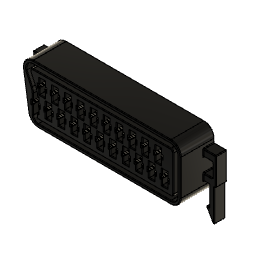
Female SCART connector ST107R-21 (Autodesk Fusion 360 design; units mm, degrees)
Autodesk Fusion 360 part; units mm, degrees
(part 1 of 2)
sketch "Sketch1" plane through (0, 0, 0) normal (0, 1, 0) x (1, 0, 0)
  line L0 (0, 0) -> (47.1, 0)
  line L1 (47.1, 0) -> (47.1, -16.5)
  line L2 (47.1, -16.5) -> (0, -16.5)
  line L3 (0, -16.5) -> (0, 0)
  line L4 (47.1, -8.25) -> (0, -8.25) construction
  line L5 (47.1, -5.71) -> (0, -5.71) construction
  line L6 (47.1, -10.79) -> (0, -10.79) construction
  line L7 (23.3, 0) -> (23.3, -16.5) construction
  line L8 (22.5, -7.81) -> (24.1, -7.81)
  line L9 (24.1, -7.81) -> (24.1, -3.61)
  line L10 (24.1, -3.61) -> (22.5, -3.61)
  line L11 (22.5, -3.61) -> (22.5, -7.81)
  line L12 (5.05, -3.61) -> (3.45, -3.61)
  line L13 (5.05, -7.81) -> (5.05, -3.61)
  line L14 (3.45, -3.61) -> (3.45, -7.81)
  line L15 (3.45, -7.81) -> (5.05, -7.81)
  line L16 (8.86, -3.61) -> (7.26, -3.61)
  line L17 (8.86, -7.81) -> (8.86, -3.61)
  line L18 (7.26, -3.61) -> (7.26, -7.81)
  line L19 (7.26, -7.81) -> (8.86, -7.81)
  line L20 (12.67, -3.61) -> (11.07, -3.61)
  line L21 (12.67, -7.81) -> (12.67, -3.61)
  line L22 (11.07, -3.61) -> (11.07, -7.81)
  line L23 (11.07, -7.81) -> (12.67, -7.81)
  line L24 (16.48, -3.61) -> (14.88, -3.61)
  line L25 (16.48, -7.81) -> (16.48, -3.61)
  line L26 (14.88, -3.61) -> (14.88, -7.81)
  line L27 (14.88, -7.81) -> (16.48, -7.81)
  line L28 (20.29, -3.61) -> (18.69, -3.61)
  line L29 (20.29, -7.81) -> (20.29, -3.61)
  line L30 (18.69, -3.61) -> (18.69, -7.81)
  line L31 (18.69, -7.81) -> (20.29, -7.81)
  line L32 (27.91, -3.61) -> (26.31, -3.61)
  line L33 (27.91, -7.81) -> (27.91, -3.61)
  line L34 (26.31, -3.61) -> (26.31, -7.81)
  line L35 (26.31, -7.81) -> (27.91, -7.81)
  line L36 (31.72, -3.61) -> (30.12, -3.61)
  line L37 (31.72, -7.81) -> (31.72, -3.61)
  line L38 (30.12, -3.61) -> (30.12, -7.81)
  line L39 (30.12, -7.81) -> (31.72, -7.81)
  line L40 (35.53, -3.61) -> (33.93, -3.61)
  line L41 (35.53, -7.81) -> (35.53, -3.61)
  line L42 (33.93, -3.61) -> (33.93, -7.81)
  line L43 (33.93, -7.81) -> (35.53, -7.81)
  line L44 (39.34, -3.61) -> (37.74, -3.61)
  line L45 (39.34, -7.81) -> (39.34, -3.61)
  line L46 (37.74, -3.61) -> (37.74, -7.81)
  line L47 (37.74, -7.81) -> (39.34, -7.81)
  line L48 (43.15, -3.61) -> (41.55, -3.61)
  line L49 (43.15, -7.81) -> (43.15, -3.61)
  line L50 (41.55, -3.61) -> (41.55, -7.81)
  line L51 (41.55, -7.81) -> (43.15, -7.81)
  line L52 (39.34, -7.81) -> (41.55, -7.81) construction
  line L53 (40.445, -7.81) -> (40.445, -14) construction
  line L54 (39.645, -12.89) -> (41.245, -12.89)
  line L55 (41.245, -12.89) -> (41.245, -8.69)
  line L56 (41.245, -8.69) -> (39.645, -8.69)
  line L57 (39.645, -8.69) -> (39.645, -12.89)
  line L58 (37.435, -12.89) -> (37.435, -8.69)
  line L59 (37.435, -8.69) -> (35.835, -8.69)
  line L60 (35.835, -8.69) -> (35.835, -12.89)
  line L61 (35.835, -12.89) -> (37.435, -12.89)
  line L62 (33.625, -12.89) -> (33.625, -8.69)
  line L63 (33.625, -8.69) -> (32.025, -8.69)
  line L64 (32.025, -8.69) -> (32.025, -12.89)
  line L65 (32.025, -12.89) -> (33.625, -12.89)
  line L66 (29.815, -12.89) -> (29.815, -8.69)
  line L67 (29.815, -8.69) -> (28.215, -8.69)
  line L68 (28.215, -8.69) -> (28.215, -12.89)
  line L69 (28.215, -12.89) -> (29.815, -12.89)
  line L70 (26.005, -12.89) -> (26.005, -8.69)
  line L71 (26.005, -8.69) -> (24.405, -8.69)
  line L72 (24.405, -8.69) -> (24.405, -12.89)
  line L73 (24.405, -12.89) -> (26.005, -12.89)
  line L74 (22.195, -12.89) -> (22.195, -8.69)
  line L75 (22.195, -8.69) -> (20.595, -8.69)
  line L76 (20.595, -8.69) -> (20.595, -12.89)
  line L77 (20.595, -12.89) -> (22.195, -12.89)
  line L78 (18.385, -12.89) -> (18.385, -8.69)
  line L79 (18.385, -8.69) -> (16.785, -8.69)
  line L80 (16.785, -8.69) -> (16.785, -12.89)
  line L81 (16.785, -12.89) -> (18.385, -12.89)
  line L82 (14.575, -12.89) -> (14.575, -8.69)
  line L83 (14.575, -8.69) -> (12.975, -8.69)
  line L84 (12.975, -8.69) -> (12.975, -12.89)
  line L85 (12.975, -12.89) -> (14.575, -12.89)
  line L86 (10.765, -12.89) -> (10.765, -8.69)
  line L87 (10.765, -8.69) -> (9.165, -8.69)
  line L88 (9.165, -8.69) -> (9.165, -12.89)
  line L89 (9.165, -12.89) -> (10.765, -12.89)
  line L90 (6.955, -12.89) -> (6.955, -8.69)
  line L91 (6.955, -8.69) -> (5.355, -8.69)
  line L92 (5.355, -8.69) -> (5.355, -12.89)
  line L93 (5.355, -12.89) -> (6.955, -12.89)
  line L94 (0, -16.5) -> (2.5, 0)
  line L95 (22.1, -6.21) -> (24.5, -6.21)
  line L96 (24.5, -6.21) -> (24.5, -5.21)
  line L97 (24.5, -5.21) -> (22.1, -5.21)
  line L98 (22.1, -5.21) -> (22.1, -6.21)
  line L99 (5.45, -5.21) -> (3.05, -5.21)
  line L100 (5.45, -6.21) -> (5.45, -5.21)
  line L101 (3.05, -6.21) -> (5.45, -6.21)
  line L102 (3.05, -5.21) -> (3.05, -6.21)
  line L103 (9.26, -5.21) -> (6.86, -5.21)
  line L104 (9.26, -6.21) -> (9.26, -5.21)
  line L105 (6.86, -6.21) -> (9.26, -6.21)
  line L106 (6.86, -5.21) -> (6.86, -6.21)
  line L107 (13.07, -5.21) -> (10.67, -5.21)
  line L108 (13.07, -6.21) -> (13.07, -5.21)
  line L109 (10.67, -6.21) -> (13.07, -6.21)
  line L110 (10.67, -5.21) -> (10.67, -6.21)
  line L111 (16.88, -5.21) -> (14.48, -5.21)
  line L112 (16.88, -6.21) -> (16.88, -5.21)
  line L113 (14.48, -6.21) -> (16.88, -6.21)
  line L114 (14.48, -5.21) -> (14.48, -6.21)
  line L115 (20.69, -5.21) -> (18.29, -5.21)
  line L116 (20.69, -6.21) -> (20.69, -5.21)
  line L117 (18.29, -6.21) -> (20.69, -6.21)
  line L118 (18.29, -5.21) -> (18.29, -6.21)
  line L119 (28.31, -5.21) -> (25.91, -5.21)
  line L120 (28.31, -6.21) -> (28.31, -5.21)
  line L121 (25.91, -6.21) -> (28.31, -6.21)
  line L122 (25.91, -5.21) -> (25.91, -6.21)
  line L123 (32.12, -5.21) -> (29.72, -5.21)
  line L124 (32.12, -6.21) -> (32.12, -5.21)
  line L125 (29.72, -6.21) -> (32.12, -6.21)
  line L126 (29.72, -5.21) -> (29.72, -6.21)
  line L127 (35.93, -5.21) -> (33.53, -5.21)
  line L128 (35.93, -6.21) -> (35.93, -5.21)
  line L129 (33.53, -6.21) -> (35.93, -6.21)
  line L130 (33.53, -5.21) -> (33.53, -6.21)
  line L131 (39.74, -5.21) -> (37.34, -5.21)
  line L132 (39.74, -6.21) -> (39.74, -5.21)
  line L133 (37.34, -6.21) -> (39.74, -6.21)
  line L134 (37.34, -5.21) -> (37.34, -6.21)
  line L135 (43.55, -5.21) -> (41.15, -5.21)
  line L136 (43.55, -6.21) -> (43.55, -5.21)
  line L137 (41.15, -6.21) -> (43.55, -6.21)
  line L138 (41.15, -5.21) -> (41.15, -6.21)
  line L139 (39.245, -11.29) -> (41.645, -11.29)
  line L140 (41.645, -11.29) -> (41.645, -10.29)
  line L141 (41.645, -10.29) -> (39.245, -10.29)
  line L142 (39.245, -10.29) -> (39.245, -11.29)
  line L143 (35.435, -11.29) -> (37.835, -11.29)
  line L144 (37.835, -10.29) -> (35.435, -10.29)
  line L145 (35.435, -10.29) -> (35.435, -11.29)
  line L146 (37.835, -11.29) -> (37.835, -10.29)
  line L147 (31.625, -11.29) -> (34.025, -11.29)
  line L148 (34.025, -10.29) -> (31.625, -10.29)
  line L149 (31.625, -10.29) -> (31.625, -11.29)
  line L150 (34.025, -11.29) -> (34.025, -10.29)
  line L151 (27.815, -11.29) -> (30.215, -11.29)
  line L152 (30.215, -10.29) -> (27.815, -10.29)
  line L153 (27.815, -10.29) -> (27.815, -11.29)
  line L154 (30.215, -11.29) -> (30.215, -10.29)
  line L155 (24.005, -11.29) -> (26.405, -11.29)
  line L156 (26.405, -10.29) -> (24.005, -10.29)
  line L157 (24.005, -10.29) -> (24.005, -11.29)
  line L158 (26.405, -11.29) -> (26.405, -10.29)
  line L159 (20.195, -11.29) -> (22.595, -11.29)
  line L160 (22.595, -10.29) -> (20.195, -10.29)
  line L161 (20.195, -10.29) -> (20.195, -11.29)
  line L162 (22.595, -11.29) -> (22.595, -10.29)
  line L163 (16.385, -11.29) -> (18.785, -11.29)
  line L164 (18.785, -10.29) -> (16.385, -10.29)
  line L165 (16.385, -10.29) -> (16.385, -11.29)
  line L166 (18.785, -11.29) -> (18.785, -10.29)
  line L167 (12.575, -11.29) -> (14.975, -11.29)
  line L168 (14.975, -10.29) -> (12.575, -10.29)
  line L169 (12.575, -10.29) -> (12.575, -11.29)
  line L170 (14.975, -11.29) -> (14.975, -10.29)
  line L171 (8.765, -11.29) -> (11.165, -11.29)
  line L172 (11.165, -10.29) -> (8.765, -10.29)
  line L173 (8.765, -10.29) -> (8.765, -11.29)
  line L174 (11.165, -11.29) -> (11.165, -10.29)
  line L175 (4.955, -11.29) -> (7.355, -11.29)
  line L176 (7.355, -10.29) -> (4.955, -10.29)
  line L177 (4.955, -10.29) -> (4.955, -11.29)
  line L178 (7.355, -11.29) -> (7.355, -10.29)
  dimension "d15" = 47.1
  dimension "d16" = 16.5
  dimension "d19" = 5.08
  dimension "d20" = 23.8
  dimension "d21" = 1.6
  dimension "d22" = 4.2
  dimension "d25" = 3.81
  dimension "d26" = 0
  dimension "d27" = 4.2
  dimension "d28" = 1.6
  dimension "d31" = -3.81
  dimension "d32" = 0
  dimension "d36" = 1
  dimension "d37" = 2.4
  dimension "d38" = 2.4
  dimension "d39" = 1
  constraint horizontal L0
  constraint vertical L1
  constraint horizontal L2
  constraint vertical L3
  constraint coincident L0.start L3.end
  constraint midpoint L1 L4.start
  constraint midpoint L3 L4.end
  constraint parallel L4 L5
  constraint parallel L4 L6
  constraint symmetric L4 L5 L6
  constraint horizontal L8
  constraint vertical L9
  constraint horizontal L10
  constraint vertical L11
  constraint symmetric L5 L8 L10
  constraint symmetric L7 L9 L11
  constraint midpoint L52 L53.start
  constraint perpendicular L6 L53
  constraint horizontal L54
  constraint vertical L55
  constraint horizontal L56
  constraint vertical L57
  constraint symmetric L53 L55 L57
  constraint symmetric L6 L54 L56
  constraint coincident L0 L94.end
  constraint horizontal L95
  constraint vertical L96
  constraint horizontal L97
  constraint vertical L98
  constraint symmetric L7 L96 L98
  constraint symmetric L5 L95 L97
  constraint horizontal L139
  constraint vertical L140
  constraint horizontal L141
  constraint vertical L142
  constraint symmetric L53 L140 L142
  constraint symmetric L6 L139 L141
  measures "d15" distance of L0.start L0.end
  measures "d16" distance of L0.start L2.end
  measures "d19" distance of L5 L6
  measures "d21" distance of L8.start L8.end
  measures "d22" distance of L8.start L10.end
  measures "d27" distance of L54.end L55.end
  measures "d28" distance of L54.start L54.end
  measures "d36" distance of L95.end L96.end
  measures "d37" distance of L95.start L95.end
  measures "d38" distance of L139.start L139.end
  measures "d39" distance of L139.start L141.end
extrude "Extrude4" add sketch "Sketch1" along normal blind 10 contours L0 L1 L2 L94 makes body 1
fillet "Fillet3" radius 3 4 edges at (47.1, 5, 16.5) (47.1, 5, 0) (0, 5, 16.5) (2.5, 5, 0) on bodies 1
sketch "Sketch4" plane through (0, 0, 0) normal (0, -1, 0) x (1, 0, 0)
  line L0 (26.405, 11.29) -> (26.405, 10.29)
  line L1 (26.405, 10.29) -> (26.005, 10.29)
  line L2 (26.005, 10.29) -> (26.005, 8.69)
  line L3 (26.005, 8.69) -> (24.405, 8.69)
  line L4 (24.405, 8.69) -> (24.405, 10.29)
  line L5 (24.405, 10.29) -> (24.005, 10.29)
  line L6 (24.005, 10.29) -> (24.005, 11.29)
  line L7 (24.005, 11.29) -> (24.405, 11.29)
  line L8 (24.405, 11.29) -> (24.405, 12.89)
  line L9 (24.405, 12.89) -> (26.005, 12.89)
  line L10 (26.005, 12.89) -> (26.005, 11.29)
  line L11 (26.005, 11.29) -> (26.405, 11.29)
  line L12 (22.595, 11.29) -> (22.595, 10.29)
  line L13 (22.595, 10.29) -> (22.195, 10.29)
  line L14 (22.195, 10.29) -> (22.195, 8.69)
  line L15 (22.195, 8.69) -> (20.595, 8.69)
  line L16 (20.595, 8.69) -> (20.595, 10.29)
  line L17 (20.595, 10.29) -> (20.195, 10.29)
  line L18 (20.195, 10.29) -> (20.195, 11.29)
  line L19 (20.195, 11.29) -> (20.595, 11.29)
  line L20 (20.595, 11.29) -> (20.595, 12.89)
  line L21 (20.595, 12.89) -> (22.195, 12.89)
  line L22 (22.195, 12.89) -> (22.195, 11.29)
  line L23 (22.195, 11.29) -> (22.595, 11.29)
  line L24 (11.165, 11.29) -> (11.165, 10.29)
  line L25 (11.165, 10.29) -> (10.765, 10.29)
  line L26 (10.765, 10.29) -> (10.765, 8.69)
  line L27 (10.765, 8.69) -> (9.165, 8.69)
  line L28 (9.165, 8.69) -> (9.165, 10.29)
  line L29 (9.165, 10.29) -> (8.765, 10.29)
  line L30 (8.765, 10.29) -> (8.765, 11.29)
  line L31 (8.765, 11.29) -> (9.165, 11.29)
  line L32 (9.165, 11.29) -> (9.165, 12.89)
  line L33 (9.165, 12.89) -> (10.765, 12.89)
  line L34 (10.765, 12.89) -> (10.765, 11.29)
  line L35 (10.765, 11.29) -> (11.165, 11.29)
  line L36 (39.245, 10.29) -> (39.245, 11.29)
  line L37 (39.245, 11.29) -> (39.645, 11.29)
  line L38 (39.645, 11.29) -> (39.645, 12.89)
  line L39 (39.645, 12.89) -> (41.245, 12.89)
  line L40 (41.245, 12.89) -> (41.245, 11.29)
  line L41 (41.245, 11.29) -> (41.645, 11.29)
  line L42 (41.645, 11.29) -> (41.645, 10.29)
  line L43 (41.645, 10.29) -> (41.245, 10.29)
  line L44 (41.245, 10.29) -> (41.245, 8.69)
  line L45 (41.245, 8.69) -> (39.645, 8.69)
  line L46 (39.645, 8.69) -> (39.645, 10.29)
  line L47 (39.645, 10.29) -> (39.245, 10.29)
  line L48 (37.34, 5.21) -> (37.34, 6.21)
  line L49 (37.34, 6.21) -> (37.74, 6.21)
  line L50 (37.74, 6.21) -> (37.74, 7.81)
  line L51 (37.74, 7.81) -> (39.34, 7.81)
  line L52 (39.34, 7.81) -> (39.34, 6.21)
  line L53 (39.34, 6.21) -> (39.74, 6.21)
  line L54 (39.74, 6.21) -> (39.74, 5.21)
  line L55 (39.74, 5.21) -> (39.34, 5.21)
  line L56 (39.34, 5.21) -> (39.34, 3.61)
  line L57 (39.34, 3.61) -> (37.74, 3.61)
  line L58 (37.74, 3.61) -> (37.74, 5.21)
  line L59 (37.74, 5.21) -> (37.34, 5.21)
  line L60 (3.05, 5.21) -> (3.05, 6.21)
  line L61 (3.05, 6.21) -> (3.45, 6.21)
  line L62 (3.45, 6.21) -> (3.45, 7.81)
  line L63 (3.45, 7.81) -> (5.05, 7.81)
  line L64 (5.05, 7.81) -> (5.05, 6.21)
  line L65 (5.05, 6.21) -> (5.45, 6.21)
  line L66 (5.45, 6.21) -> (5.45, 5.21)
  line L67 (5.45, 5.21) -> (5.05, 5.21)
  line L68 (5.05, 5.21) -> (5.05, 3.61)
  line L69 (5.05, 3.61) -> (3.45, 3.61)
  line L70 (3.45, 3.61) -> (3.45, 5.21)
  line L71 (3.45, 5.21) -> (3.05, 5.21)
  line L72 (6.86, 5.21) -> (6.86, 6.21)
  line L73 (6.86, 6.21) -> (7.26, 6.21)
  line L74 (7.26, 6.21) -> (7.26, 7.81)
  line L75 (7.26, 7.81) -> (8.86, 7.81)
  line L76 (8.86, 7.81) -> (8.86, 6.21)
  line L77 (8.86, 6.21) -> (9.26, 6.21)
  line L78 (9.26, 6.21) -> (9.26, 5.21)
  line L79 (9.26, 5.21) -> (8.86, 5.21)
  line L80 (8.86, 5.21) -> (8.86, 3.61)
  line L81 (8.86, 3.61) -> (7.26, 3.61)
  line L82 (7.26, 3.61) -> (7.26, 5.21)
  line L83 (7.26, 5.21) -> (6.86, 5.21)
  line L84 (10.67, 5.21) -> (10.67, 6.21)
  line L85 (10.67, 6.21) -> (11.07, 6.21)
  line L86 (11.07, 6.21) -> (11.07, 7.81)
  line L87 (11.07, 7.81) -> (12.67, 7.81)
  line L88 (12.67, 7.81) -> (12.67, 6.21)
  line L89 (12.67, 6.21) -> (13.07, 6.21)
  line L90 (13.07, 6.21) -> (13.07, 5.21)
  line L91 (13.07, 5.21) -> (12.67, 5.21)
  line L92 (12.67, 5.21) -> (12.67, 3.61)
  line L93 (12.67, 3.61) -> (11.07, 3.61)
  line L94 (11.07, 3.61) -> (11.07, 5.21)
  line L95 (11.07, 5.21) -> (10.67, 5.21)
  line L96 (30.215, 11.29) -> (30.215, 10.29)
  line L97 (30.215, 10.29) -> (29.815, 10.29)
  line L98 (29.815, 10.29) -> (29.815, 8.69)
  line L99 (29.815, 8.69) -> (28.215, 8.69)
  line L100 (28.215, 8.69) -> (28.215, 10.29)
  line L101 (28.215, 10.29) -> (27.815, 10.29)
  line L102 (27.815, 10.29) -> (27.815, 11.29)
  line L103 (27.815, 11.29) -> (28.215, 11.29)
  line L104 (28.215, 11.29) -> (28.215, 12.89)
  line L105 (28.215, 12.89) -> (29.815, 12.89)
  line L106 (29.815, 12.89) -> (29.815, 11.29)
  line L107 (29.815, 11.29) -> (30.215, 11.29)
  line L108 (18.785, 11.29) -> (18.785, 10.29)
  line L109 (18.785, 10.29) -> (18.385, 10.29)
  line L110 (18.385, 10.29) -> (18.385, 8.69)
  line L111 (18.385, 8.69) -> (16.785, 8.69)
  line L112 (16.785, 8.69) -> (16.785, 10.29)
  line L113 (16.785, 10.29) -> (16.385, 10.29)
  line L114 (16.385, 10.29) -> (16.385, 11.29)
  line L115 (16.385, 11.29) -> (16.785, 11.29)
  line L116 (16.785, 11.29) -> (16.785, 12.89)
  line L117 (16.785, 12.89) -> (18.385, 12.89)
  line L118 (18.385, 12.89) -> (18.385, 11.29)
  line L119 (18.385, 11.29) -> (18.785, 11.29)
  line L120 (14.975, 11.29) -> (14.975, 10.29)
  line L121 (14.975, 10.29) -> (14.575, 10.29)
  line L122 (14.575, 10.29) -> (14.575, 8.69)
  line L123 (14.575, 8.69) -> (12.975, 8.69)
  line L124 (12.975, 8.69) -> (12.975, 10.29)
  line L125 (12.975, 10.29) -> (12.575, 10.29)
  line L126 (12.575, 10.29) -> (12.575, 11.29)
  line L127 (12.575, 11.29) -> (12.975, 11.29)
  line L128 (12.975, 11.29) -> (12.975, 12.89)
  line L129 (12.975, 12.89) -> (14.575, 12.89)
  line L130 (14.575, 12.89) -> (14.575, 11.29)
  line L131 (14.575, 11.29) -> (14.975, 11.29)
  line L132 (34.025, 11.29) -> (34.025, 10.29)
  line L133 (34.025, 10.29) -> (33.625, 10.29)
  line L134 (33.625, 10.29) -> (33.625, 8.69)
  line L135 (33.625, 8.69) -> (32.025, 8.69)
  line L136 (32.025, 8.69) -> (32.025, 10.29)
  line L137 (32.025, 10.29) -> (31.625, 10.29)
  line L138 (31.625, 10.29) -> (31.625, 11.29)
  line L139 (31.625, 11.29) -> (32.025, 11.29)
  line L140 (32.025, 11.29) -> (32.025, 12.89)
  line L141 (32.025, 12.89) -> (33.625, 12.89)
  line L142 (33.625, 12.89) -> (33.625, 11.29)
  line L143 (33.625, 11.29) -> (34.025, 11.29)
  line L144 (25.91, 5.21) -> (25.91, 6.21)
  line L145 (25.91, 6.21) -> (26.31, 6.21)
  line L146 (26.31, 6.21) -> (26.31, 7.81)
  line L147 (26.31, 7.81) -> (27.91, 7.81)
  line L148 (27.91, 7.81) -> (27.91, 6.21)
  line L149 (27.91, 6.21) -> (28.31, 6.21)
  line L150 (28.31, 6.21) -> (28.31, 5.21)
  line L151 (28.31, 5.21) -> (27.91, 5.21)
  line L152 (27.91, 5.21) -> (27.91, 3.61)
  line L153 (27.91, 3.61) -> (26.31, 3.61)
  line L154 (26.31, 3.61) -> (26.31, 5.21)
  line L155 (26.31, 5.21) -> (25.91, 5.21)
  line L156 (18.29, 5.21) -> (18.29, 6.21)
  line L157 (18.29, 6.21) -> (18.69, 6.21)
  line L158 (18.69, 6.21) -> (18.69, 7.81)
  line L159 (18.69, 7.81) -> (20.29, 7.81)
  line L160 (20.29, 7.81) -> (20.29, 6.21)
  line L161 (20.29, 6.21) -> (20.69, 6.21)
  line L162 (20.69, 6.21) -> (20.69, 5.21)
  line L163 (20.69, 5.21) -> (20.29, 5.21)
  line L164 (20.29, 5.21) -> (20.29, 3.61)
  line L165 (20.29, 3.61) -> (18.69, 3.61)
  line L166 (18.69, 3.61) -> (18.69, 5.21)
  line L167 (18.69, 5.21) -> (18.29, 5.21)
  line L168 (33.53, 5.21) -> (33.53, 6.21)
  line L169 (33.53, 6.21) -> (33.93, 6.21)
  line L170 (33.93, 6.21) -> (33.93, 7.81)
  line L171 (33.93, 7.81) -> (35.53, 7.81)
  line L172 (35.53, 7.81) -> (35.53, 6.21)
  line L173 (35.53, 6.21) -> (35.93, 6.21)
  line L174 (35.93, 6.21) -> (35.93, 5.21)
  line L175 (35.93, 5.21) -> (35.53, 5.21)
  line L176 (35.53, 5.21) -> (35.53, 3.61)
  line L177 (35.53, 3.61) -> (33.93, 3.61)
  line L178 (33.93, 3.61) -> (33.93, 5.21)
  line L179 (33.93, 5.21) -> (33.53, 5.21)
  line L180 (41.15, 5.21) -> (41.15, 6.21)
  line L181 (41.15, 6.21) -> (41.55, 6.21)
  line L182 (41.55, 6.21) -> (41.55, 7.81)
  line L183 (41.55, 7.81) -> (43.15, 7.81)
  line L184 (43.15, 7.81) -> (43.15, 6.21)
  line L185 (43.15, 6.21) -> (43.55, 6.21)
  line L186 (43.55, 6.21) -> (43.55, 5.21)
  line L187 (43.55, 5.21) -> (43.15, 5.21)
  line L188 (43.15, 5.21) -> (43.15, 3.61)
  line L189 (43.15, 3.61) -> (41.55, 3.61)
  line L190 (41.55, 3.61) -> (41.55, 5.21)
  line L191 (41.55, 5.21) -> (41.15, 5.21)
  line L192 (14.48, 5.21) -> (14.48, 6.21)
  line L193 (14.48, 6.21) -> (14.88, 6.21)
  line L194 (14.88, 6.21) -> (14.88, 7.81)
  line L195 (14.88, 7.81) -> (16.48, 7.81)
  line L196 (16.48, 7.81) -> (16.48, 6.21)
  line L197 (16.48, 6.21) -> (16.88, 6.21)
  line L198 (16.88, 6.21) -> (16.88, 5.21)
  line L199 (16.88, 5.21) -> (16.48, 5.21)
  line L200 (16.48, 5.21) -> (16.48, 3.61)
  line L201 (16.48, 3.61) -> (14.88, 3.61)
  line L202 (14.88, 3.61) -> (14.88, 5.21)
  line L203 (14.88, 5.21) -> (14.48, 5.21)
  line L204 (37.835, 11.29) -> (37.835, 10.29)
  line L205 (37.835, 10.29) -> (37.435, 10.29)
  line L206 (37.435, 10.29) -> (37.435, 8.69)
  line L207 (37.435, 8.69) -> (35.835, 8.69)
  line L208 (35.835, 8.69) -> (35.835, 10.29)
  line L209 (35.835, 10.29) -> (35.435, 10.29)
  line L210 (35.435, 10.29) -> (35.435, 11.29)
  line L211 (35.435, 11.29) -> (35.835, 11.29)
  line L212 (35.835, 11.29) -> (35.835, 12.89)
  line L213 (35.835, 12.89) -> (37.435, 12.89)
  line L214 (37.435, 12.89) -> (37.435, 11.29)
  line L215 (37.435, 11.29) -> (37.835, 11.29)
  line L216 (7.355, 11.29) -> (7.355, 10.29)
  line L217 (7.355, 10.29) -> (6.955, 10.29)
  line L218 (6.955, 10.29) -> (6.955, 8.69)
  line L219 (6.955, 8.69) -> (5.355, 8.69)
  line L220 (5.355, 8.69) -> (5.355, 10.29)
  line L221 (5.355, 10.29) -> (4.955, 10.29)
  line L222 (4.955, 10.29) -> (4.955, 11.29)
  line L223 (4.955, 11.29) -> (5.355, 11.29)
  line L224 (5.355, 11.29) -> (5.355, 12.89)
  line L225 (5.355, 12.89) -> (6.955, 12.89)
  line L226 (6.955, 12.89) -> (6.955, 11.29)
  line L227 (6.955, 11.29) -> (7.355, 11.29)
  line L228 (29.72, 5.21) -> (29.72, 6.21)
  line L229 (29.72, 6.21) -> (30.12, 6.21)
  line L230 (30.12, 6.21) -> (30.12, 7.81)
  line L231 (30.12, 7.81) -> (31.72, 7.81)
  line L232 (31.72, 7.81) -> (31.72, 6.21)
  line L233 (31.72, 6.21) -> (32.12, 6.21)
  line L234 (32.12, 6.21) -> (32.12, 5.21)
  line L235 (32.12, 5.21) -> (31.72, 5.21)
  line L236 (31.72, 5.21) -> (31.72, 3.61)
  line L237 (31.72, 3.61) -> (30.12, 3.61)
  line L238 (30.12, 3.61) -> (30.12, 5.21)
  line L239 (30.12, 5.21) -> (29.72, 5.21)
  line L240 (22.1, 5.21) -> (22.1, 6.21)
  line L241 (22.1, 6.21) -> (22.5, 6.21)
  line L242 (22.5, 6.21) -> (22.5, 7.81)
  line L243 (22.5, 7.81) -> (24.1, 7.81)
  line L244 (24.1, 7.81) -> (24.1, 6.21)
  line L245 (24.1, 6.21) -> (24.5, 6.21)
  line L246 (24.5, 6.21) -> (24.5, 5.21)
  line L247 (24.5, 5.21) -> (24.1, 5.21)
  line L248 (24.1, 5.21) -> (24.1, 3.61)
  line L249 (24.1, 3.61) -> (22.5, 3.61)
  line L250 (22.5, 3.61) -> (22.5, 5.21)
  line L251 (22.5, 5.21) -> (22.1, 5.21)
  arc A0 (2.1135, 2.5506) -> (5.0797, 0) centre (5.0797, 3) ccw
  line L252 (5.0797, 0) -> (44.1, 0)
  arc A1 (44.1, 0) -> (47.1, 3) centre (44.1, 3) ccw
  line L253 (47.1, 3) -> (47.1, 13.5)
  arc A2 (47.1, 13.5) -> (44.1, 16.5) centre (44.1, 13.5) ccw
  line L254 (44.1, 16.5) -> (3.4888, 16.5)
  arc A3 (3.4888, 16.5) -> (0.5226, 13.0506) centre (3.4888, 13.5) ccw
  line L255 (0.5226, 13.0506) -> (2.1135, 2.5506)
  line L256 (4.95, 0.9759) -> (44.1, 0.9759)
  arc A4 (44.1, 0.9759) -> (46.1241, 3) centre (44.1, 3) ccw
  line L257 (46.1241, 3) -> (46.1241, 13.5)
  arc A5 (46.1241, 13.5) -> (44.1, 15.5241) centre (44.1, 13.5) ccw
  line L258 (44.1, 15.5241) -> (3.4888, 15.5241)
  arc A6 (3.4888, 15.5241) -> (1.5281, 12.9976) centre (3.4888, 13.5) ccw
  line L259 (3.45, 3.61) -> (3.45, 2.4759)
  arc A7 (3.45, 2.4759) -> (4.95, 0.9759) centre (4.95, 2.4759) ccw
  line L260 (3.45, 7.81) -> (3.45, 8.0452)
  line L261 (3.131, 9.5051) -> (1.5281, 12.9976)
  arc A8 (3.45, 8.0452) -> (3.131, 9.5051) centre (-0.05, 8.0452) ccw
  line L262 (4.65, 3.61) -> (4.65, 2.4759)
  arc A9 (4.65, 2.4759) -> (4.95, 2.1759) centre (4.95, 2.4759) ccw
  line L263 (4.95, 2.1759) -> (44.1, 2.1759)
  arc A10 (44.1, 2.1759) -> (44.9241, 3) centre (44.1, 3) ccw
  line L264 (44.9241, 3) -> (44.9241, 13.5)
  arc A11 (44.9241, 13.5) -> (44.1, 14.3241) centre (44.1, 13.5) ccw
  line L265 (44.1, 14.3241) -> (3.4888, 14.3241)
  arc A12 (3.4888, 14.3241) -> (2.6738, 13.3781) centre (3.4888, 13.5) ccw
  line L266 (4.2216, 10.0057) -> (2.6738, 13.3781)
  arc A13 (4.65, 8.0452) -> (4.2216, 10.0057) centre (-0.05, 8.0452) ccw
  line L267 (4.65, 7.81) -> (4.65, 8.0452)
  point P0 (3.45, 8.81)
  dimension "d41" = 1.5
  dimension "d42" = 1
  dimension "d43" = 3.5
  dimension "d44" = -1.2
  constraint coincident L69.end L70.start
  constraint perpendicular L69 L259
  constraint parallel L252 L256
  constraint concentric A1 A4
  constraint parallel L253 L257
  constraint concentric A2 A5
  constraint parallel L254 L258
  constraint concentric A3 A6
  constraint tangent L258 A6
  constraint tangent L257 A5
  constraint tangent L256 A4
  constraint tangent A5 L258
  constraint tangent A4 L257
  constraint tangent L259 A7
  constraint tangent L256 A7
  constraint coincident L62.end L63.start
  constraint perpendicular L63 L260
  constraint coincident P0 L260
  constraint coincident P0 L261
  constraint tangent L260 A8
  constraint tangent L261 A8
  measures "d41" radius of A7
  measures "d42" distance of L62.end P0
  measures "d43" radius of A8
extrude "Extrude5" cut sketch "Sketch4" against normal blind 8 contours L63 L69 L256 A4 L257 A5 L258 A6 L259 A7 L260 L261 A8 L262 A9 L263 A10 L264 A11 L265 A12 L266 A13 L267 bodies 1
sketch "Sketch5" plane through (0, 10, 0) normal (0, 1, 0) x (-1, 0, 0)
  arc A0 (-5.0797, 0) -> (-2.1135, 2.5506) centre (-5.0797, 3) ccw
  line L0 (-2.1135, 2.5506) -> (-0.5226, 13.0506)
  arc A1 (-0.5226, 13.0506) -> (-3.4888, 16.5) centre (-3.4888, 13.5) ccw
  line L1 (-3.4888, 16.5) -> (-44.1, 16.5)
  arc A2 (-44.1, 16.5) -> (-47.1, 13.5) centre (-44.1, 13.5) ccw
  line L2 (-47.1, 13.5) -> (-47.1, 3)
  arc A3 (-47.1, 3) -> (-44.1, 0) centre (-44.1, 3) ccw
  line L3 (-44.1, 0) -> (-5.0797, 0)
  line L4 (-26.405, 10.29) -> (-26.405, 11.29)
  line L5 (-26.405, 11.29) -> (-26.005, 11.29)
  line L6 (-26.005, 11.29) -> (-26.005, 12.89)
  line L7 (-26.005, 12.89) -> (-24.405, 12.89)
  line L8 (-24.405, 12.89) -> (-24.405, 11.29)
  line L9 (-24.405, 11.29) -> (-24.005, 11.29)
  line L10 (-24.005, 11.29) -> (-24.005, 10.29)
  line L11 (-24.005, 10.29) -> (-24.405, 10.29)
  line L12 (-24.405, 10.29) -> (-24.405, 8.69)
  line L13 (-24.405, 8.69) -> (-26.005, 8.69)
  line L14 (-26.005, 8.69) -> (-26.005, 10.29)
  line L15 (-26.005, 10.29) -> (-26.405, 10.29)
  line L16 (-22.595, 10.29) -> (-22.595, 11.29)
  line L17 (-22.595, 11.29) -> (-22.195, 11.29)
  line L18 (-22.195, 11.29) -> (-22.195, 12.89)
  line L19 (-22.195, 12.89) -> (-20.595, 12.89)
  line L20 (-20.595, 12.89) -> (-20.595, 11.29)
  line L21 (-20.595, 11.29) -> (-20.195, 11.29)
  line L22 (-20.195, 11.29) -> (-20.195, 10.29)
  line L23 (-20.195, 10.29) -> (-20.595, 10.29)
  line L24 (-20.595, 10.29) -> (-20.595, 8.69)
  line L25 (-20.595, 8.69) -> (-22.195, 8.69)
  line L26 (-22.195, 8.69) -> (-22.195, 10.29)
  line L27 (-22.195, 10.29) -> (-22.595, 10.29)
  line L28 (-11.165, 10.29) -> (-11.165, 11.29)
  line L29 (-11.165, 11.29) -> (-10.765, 11.29)
  line L30 (-10.765, 11.29) -> (-10.765, 12.89)
  line L31 (-10.765, 12.89) -> (-9.165, 12.89)
  line L32 (-9.165, 12.89) -> (-9.165, 11.29)
  line L33 (-9.165, 11.29) -> (-8.765, 11.29)
  line L34 (-8.765, 11.29) -> (-8.765, 10.29)
  line L35 (-8.765, 10.29) -> (-9.165, 10.29)
  line L36 (-9.165, 10.29) -> (-9.165, 8.69)
  line L37 (-9.165, 8.69) -> (-10.765, 8.69)
  line L38 (-10.765, 8.69) -> (-10.765, 10.29)
  line L39 (-10.765, 10.29) -> (-11.165, 10.29)
  line L40 (-39.245, 11.29) -> (-39.245, 10.29)
  line L41 (-39.245, 10.29) -> (-39.645, 10.29)
  line L42 (-39.645, 10.29) -> (-39.645, 8.69)
  line L43 (-39.645, 8.69) -> (-41.245, 8.69)
  line L44 (-41.245, 8.69) -> (-41.245, 10.29)
  line L45 (-41.245, 10.29) -> (-41.645, 10.29)
  line L46 (-41.645, 10.29) -> (-41.645, 11.29)
  line L47 (-41.645, 11.29) -> (-41.245, 11.29)
  line L48 (-41.245, 11.29) -> (-41.245, 12.89)
  line L49 (-41.245, 12.89) -> (-39.645, 12.89)
  line L50 (-39.645, 12.89) -> (-39.645, 11.29)
  line L51 (-39.645, 11.29) -> (-39.245, 11.29)
  line L52 (-37.34, 6.21) -> (-37.34, 5.21)
  line L53 (-37.34, 5.21) -> (-37.74, 5.21)
  line L54 (-37.74, 5.21) -> (-37.74, 3.61)
  line L55 (-37.74, 3.61) -> (-39.34, 3.61)
  line L56 (-39.34, 3.61) -> (-39.34, 5.21)
  line L57 (-39.34, 5.21) -> (-39.74, 5.21)
  line L58 (-39.74, 5.21) -> (-39.74, 6.21)
  line L59 (-39.74, 6.21) -> (-39.34, 6.21)
  line L60 (-39.34, 6.21) -> (-39.34, 7.81)
  line L61 (-39.34, 7.81) -> (-37.74, 7.81)
  line L62 (-37.74, 7.81) -> (-37.74, 6.21)
  line L63 (-37.74, 6.21) -> (-37.34, 6.21)
  line L64 (-3.05, 6.21) -> (-3.05, 5.21)
  line L65 (-3.05, 5.21) -> (-3.45, 5.21)
  line L66 (-3.45, 5.21) -> (-3.45, 3.61)
  line L67 (-3.45, 3.61) -> (-5.05, 3.61)
  line L68 (-5.05, 3.61) -> (-5.05, 5.21)
  line L69 (-5.05, 5.21) -> (-5.45, 5.21)
  line L70 (-5.45, 5.21) -> (-5.45, 6.21)
  line L71 (-5.45, 6.21) -> (-5.05, 6.21)
  line L72 (-5.05, 6.21) -> (-5.05, 7.81)
  line L73 (-5.05, 7.81) -> (-3.45, 7.81)
  line L74 (-3.45, 7.81) -> (-3.45, 6.21)
  line L75 (-3.45, 6.21) -> (-3.05, 6.21)
  line L76 (-6.86, 6.21) -> (-6.86, 5.21)
  line L77 (-6.86, 5.21) -> (-7.26, 5.21)
  line L78 (-7.26, 5.21) -> (-7.26, 3.61)
  line L79 (-7.26, 3.61) -> (-8.86, 3.61)
  line L80 (-8.86, 3.61) -> (-8.86, 5.21)
  line L81 (-8.86, 5.21) -> (-9.26, 5.21)
  line L82 (-9.26, 5.21) -> (-9.26, 6.21)
  line L83 (-9.26, 6.21) -> (-8.86, 6.21)
  line L84 (-8.86, 6.21) -> (-8.86, 7.81)
  line L85 (-8.86, 7.81) -> (-7.26, 7.81)
  line L86 (-7.26, 7.81) -> (-7.26, 6.21)
  line L87 (-7.26, 6.21) -> (-6.86, 6.21)
  line L88 (-10.67, 6.21) -> (-10.67, 5.21)
  line L89 (-10.67, 5.21) -> (-11.07, 5.21)
  line L90 (-11.07, 5.21) -> (-11.07, 3.61)
  line L91 (-11.07, 3.61) -> (-12.67, 3.61)
  line L92 (-12.67, 3.61) -> (-12.67, 5.21)
  line L93 (-12.67, 5.21) -> (-13.07, 5.21)
  line L94 (-13.07, 5.21) -> (-13.07, 6.21)
  line L95 (-13.07, 6.21) -> (-12.67, 6.21)
  line L96 (-12.67, 6.21) -> (-12.67, 7.81)
  line L97 (-12.67, 7.81) -> (-11.07, 7.81)
  line L98 (-11.07, 7.81) -> (-11.07, 6.21)
  line L99 (-11.07, 6.21) -> (-10.67, 6.21)
  line L100 (-30.215, 10.29) -> (-30.215, 11.29)
  line L101 (-30.215, 11.29) -> (-29.815, 11.29)
  line L102 (-29.815, 11.29) -> (-29.815, 12.89)
  line L103 (-29.815, 12.89) -> (-28.215, 12.89)
  line L104 (-28.215, 12.89) -> (-28.215, 11.29)
  line L105 (-28.215, 11.29) -> (-27.815, 11.29)
  line L106 (-27.815, 11.29) -> (-27.815, 10.29)
  line L107 (-27.815, 10.29) -> (-28.215, 10.29)
  line L108 (-28.215, 10.29) -> (-28.215, 8.69)
  line L109 (-28.215, 8.69) -> (-29.815, 8.69)
  line L110 (-29.815, 8.69) -> (-29.815, 10.29)
  line L111 (-29.815, 10.29) -> (-30.215, 10.29)
  line L112 (-18.785, 10.29) -> (-18.785, 11.29)
  line L113 (-18.785, 11.29) -> (-18.385, 11.29)
  line L114 (-18.385, 11.29) -> (-18.385, 12.89)
  line L115 (-18.385, 12.89) -> (-16.785, 12.89)
  line L116 (-16.785, 12.89) -> (-16.785, 11.29)
  line L117 (-16.785, 11.29) -> (-16.385, 11.29)
  line L118 (-16.385, 11.29) -> (-16.385, 10.29)
  line L119 (-16.385, 10.29) -> (-16.785, 10.29)
  line L120 (-16.785, 10.29) -> (-16.785, 8.69)
  line L121 (-16.785, 8.69) -> (-18.385, 8.69)
  line L122 (-18.385, 8.69) -> (-18.385, 10.29)
  line L123 (-18.385, 10.29) -> (-18.785, 10.29)
  line L124 (-14.975, 10.29) -> (-14.975, 11.29)
  line L125 (-14.975, 11.29) -> (-14.575, 11.29)
  line L126 (-14.575, 11.29) -> (-14.575, 12.89)
  line L127 (-14.575, 12.89) -> (-12.975, 12.89)
  line L128 (-12.975, 12.89) -> (-12.975, 11.29)
  line L129 (-12.975, 11.29) -> (-12.575, 11.29)
  line L130 (-12.575, 11.29) -> (-12.575, 10.29)
  line L131 (-12.575, 10.29) -> (-12.975, 10.29)
  line L132 (-12.975, 10.29) -> (-12.975, 8.69)
  line L133 (-12.975, 8.69) -> (-14.575, 8.69)
  line L134 (-14.575, 8.69) -> (-14.575, 10.29)
  line L135 (-14.575, 10.29) -> (-14.975, 10.29)
  line L136 (-34.025, 10.29) -> (-34.025, 11.29)
  line L137 (-34.025, 11.29) -> (-33.625, 11.29)
  line L138 (-33.625, 11.29) -> (-33.625, 12.89)
  line L139 (-33.625, 12.89) -> (-32.025, 12.89)
  line L140 (-32.025, 12.89) -> (-32.025, 11.29)
  line L141 (-32.025, 11.29) -> (-31.625, 11.29)
  line L142 (-31.625, 11.29) -> (-31.625, 10.29)
  line L143 (-31.625, 10.29) -> (-32.025, 10.29)
  line L144 (-32.025, 10.29) -> (-32.025, 8.69)
  line L145 (-32.025, 8.69) -> (-33.625, 8.69)
  line L146 (-33.625, 8.69) -> (-33.625, 10.29)
  line L147 (-33.625, 10.29) -> (-34.025, 10.29)
  line L148 (-25.91, 6.21) -> (-25.91, 5.21)
  line L149 (-25.91, 5.21) -> (-26.31, 5.21)
  line L150 (-26.31, 5.21) -> (-26.31, 3.61)
  line L151 (-26.31, 3.61) -> (-27.91, 3.61)
  line L152 (-27.91, 3.61) -> (-27.91, 5.21)
  line L153 (-27.91, 5.21) -> (-28.31, 5.21)
  line L154 (-28.31, 5.21) -> (-28.31, 6.21)
  line L155 (-28.31, 6.21) -> (-27.91, 6.21)
  line L156 (-27.91, 6.21) -> (-27.91, 7.81)
  line L157 (-27.91, 7.81) -> (-26.31, 7.81)
  line L158 (-26.31, 7.81) -> (-26.31, 6.21)
  line L159 (-26.31, 6.21) -> (-25.91, 6.21)
  line L160 (-18.29, 6.21) -> (-18.29, 5.21)
  line L161 (-18.29, 5.21) -> (-18.69, 5.21)
  line L162 (-18.69, 5.21) -> (-18.69, 3.61)
  line L163 (-18.69, 3.61) -> (-20.29, 3.61)
  line L164 (-20.29, 3.61) -> (-20.29, 5.21)
  line L165 (-20.29, 5.21) -> (-20.69, 5.21)
  line L166 (-20.69, 5.21) -> (-20.69, 6.21)
  line L167 (-20.69, 6.21) -> (-20.29, 6.21)
  line L168 (-20.29, 6.21) -> (-20.29, 7.81)
  line L169 (-20.29, 7.81) -> (-18.69, 7.81)
  line L170 (-18.69, 7.81) -> (-18.69, 6.21)
  line L171 (-18.69, 6.21) -> (-18.29, 6.21)
  line L172 (-33.53, 6.21) -> (-33.53, 5.21)
  line L173 (-33.53, 5.21) -> (-33.93, 5.21)
  line L174 (-33.93, 5.21) -> (-33.93, 3.61)
  line L175 (-33.93, 3.61) -> (-35.53, 3.61)
  line L176 (-35.53, 3.61) -> (-35.53, 5.21)
  line L177 (-35.53, 5.21) -> (-35.93, 5.21)
  line L178 (-35.93, 5.21) -> (-35.93, 6.21)
  line L179 (-35.93, 6.21) -> (-35.53, 6.21)
  line L180 (-35.53, 6.21) -> (-35.53, 7.81)
  line L181 (-35.53, 7.81) -> (-33.93, 7.81)
  line L182 (-33.93, 7.81) -> (-33.93, 6.21)
  line L183 (-33.93, 6.21) -> (-33.53, 6.21)
  line L184 (-41.15, 6.21) -> (-41.15, 5.21)
  line L185 (-41.15, 5.21) -> (-41.55, 5.21)
  line L186 (-41.55, 5.21) -> (-41.55, 3.61)
  line L187 (-41.55, 3.61) -> (-43.15, 3.61)
  line L188 (-43.15, 3.61) -> (-43.15, 5.21)
  line L189 (-43.15, 5.21) -> (-43.55, 5.21)
  line L190 (-43.55, 5.21) -> (-43.55, 6.21)
  line L191 (-43.55, 6.21) -> (-43.15, 6.21)
  line L192 (-43.15, 6.21) -> (-43.15, 7.81)
  line L193 (-43.15, 7.81) -> (-41.55, 7.81)
  line L194 (-41.55, 7.81) -> (-41.55, 6.21)
  line L195 (-41.55, 6.21) -> (-41.15, 6.21)
  line L196 (-14.48, 6.21) -> (-14.48, 5.21)
  line L197 (-14.48, 5.21) -> (-14.88, 5.21)
  line L198 (-14.88, 5.21) -> (-14.88, 3.61)
  line L199 (-14.88, 3.61) -> (-16.48, 3.61)
  line L200 (-16.48, 3.61) -> (-16.48, 5.21)
  line L201 (-16.48, 5.21) -> (-16.88, 5.21)
  line L202 (-16.88, 5.21) -> (-16.88, 6.21)
  line L203 (-16.88, 6.21) -> (-16.48, 6.21)
  line L204 (-16.48, 6.21) -> (-16.48, 7.81)
  line L205 (-16.48, 7.81) -> (-14.88, 7.81)
  line L206 (-14.88, 7.81) -> (-14.88, 6.21)
  line L207 (-14.88, 6.21) -> (-14.48, 6.21)
  line L208 (-37.835, 10.29) -> (-37.835, 11.29)
  line L209 (-37.835, 11.29) -> (-37.435, 11.29)
  line L210 (-37.435, 11.29) -> (-37.435, 12.89)
  line L211 (-37.435, 12.89) -> (-35.835, 12.89)
  line L212 (-35.835, 12.89) -> (-35.835, 11.29)
  line L213 (-35.835, 11.29) -> (-35.435, 11.29)
  line L214 (-35.435, 11.29) -> (-35.435, 10.29)
  line L215 (-35.435, 10.29) -> (-35.835, 10.29)
  line L216 (-35.835, 10.29) -> (-35.835, 8.69)
  line L217 (-35.835, 8.69) -> (-37.435, 8.69)
  line L218 (-37.435, 8.69) -> (-37.435, 10.29)
  line L219 (-37.435, 10.29) -> (-37.835, 10.29)
  line L220 (-7.355, 10.29) -> (-7.355, 11.29)
  line L221 (-7.355, 11.29) -> (-6.955, 11.29)
  line L222 (-6.955, 11.29) -> (-6.955, 12.89)
  line L223 (-6.955, 12.89) -> (-5.355, 12.89)
  line L224 (-5.355, 12.89) -> (-5.355, 11.29)
  line L225 (-5.355, 11.29) -> (-4.955, 11.29)
  line L226 (-4.955, 11.29) -> (-4.955, 10.29)
  line L227 (-4.955, 10.29) -> (-5.355, 10.29)
  line L228 (-5.355, 10.29) -> (-5.355, 8.69)
  line L229 (-5.355, 8.69) -> (-6.955, 8.69)
  line L230 (-6.955, 8.69) -> (-6.955, 10.29)
  line L231 (-6.955, 10.29) -> (-7.355, 10.29)
  line L232 (-29.72, 6.21) -> (-29.72, 5.21)
  line L233 (-29.72, 5.21) -> (-30.12, 5.21)
  line L234 (-30.12, 5.21) -> (-30.12, 3.61)
  line L235 (-30.12, 3.61) -> (-31.72, 3.61)
  line L236 (-31.72, 3.61) -> (-31.72, 5.21)
  line L237 (-31.72, 5.21) -> (-32.12, 5.21)
  line L238 (-32.12, 5.21) -> (-32.12, 6.21)
  line L239 (-32.12, 6.21) -> (-31.72, 6.21)
  line L240 (-31.72, 6.21) -> (-31.72, 7.81)
  line L241 (-31.72, 7.81) -> (-30.12, 7.81)
  line L242 (-30.12, 7.81) -> (-30.12, 6.21)
  line L243 (-30.12, 6.21) -> (-29.72, 6.21)
  line L244 (-22.1, 6.21) -> (-22.1, 5.21)
  line L245 (-22.1, 5.21) -> (-22.5, 5.21)
  line L246 (-22.5, 5.21) -> (-22.5, 3.61)
  line L247 (-22.5, 3.61) -> (-24.1, 3.61)
  line L248 (-24.1, 3.61) -> (-24.1, 5.21)
  line L249 (-24.1, 5.21) -> (-24.5, 5.21)
  line L250 (-24.5, 5.21) -> (-24.5, 6.21)
  line L251 (-24.5, 6.21) -> (-24.1, 6.21)
  line L252 (-24.1, 6.21) -> (-24.1, 7.81)
  line L253 (-24.1, 7.81) -> (-22.5, 7.81)
  line L254 (-22.5, 7.81) -> (-22.5, 6.21)
  line L255 (-22.5, 6.21) -> (-22.1, 6.21)
  line L256 (-41.645, 11.29) -> (-4.955, 11.29)
  line L257 (-41.645, 10.29) -> (-4.955, 10.29)
  line L258 (-43.55, 6.21) -> (-3.05, 6.21)
  line L259 (-43.55, 5.21) -> (-3.05, 5.21)
  constraint coincident L46.end L47.start
  constraint coincident L225.end L226.start
  constraint coincident L45.end L46.start
  constraint coincident L226.end L227.start
  constraint coincident L190.end L191.start
  constraint coincident L64.start L75.end
  constraint coincident L189.end L190.start
  constraint coincident L64.end L65.start
extrude "Extrude6" add sketch "Sketch5" against normal blind 2 contours L12 L13 L14 L257 | L6 L7 L8 L256 | L108 L109 L110 L257 | L102 L103 L104 L256 | L24 L25 L26 L257 | L18 L19 L20 L256 | L144 L145 L146 L257 | L138 L139 L140 L256 | L120 L121 L122 L257 | L114 L115 L116 L256 | L216 L217 L218 L257 | L210 L211 L212 L256 | L132 L133 L134 L257 | L126 L127 L128 L256 | L42 L43 L44 L257 | L48 L49 L50 L256 | L36 L37 L38 L257 | L30 L31 L32 L256 | L228 L229 L230 L257 | L222 L223 L224 L256 | L60 L61 L62 L258 | L54 L55 L56 L259 | L180 L181 L182 L258 | L174 L175 L176 L259 | L192 L193 L194 L258 | L186 L187 L188 L259 | L240 L241 L242 L258 | L234 L235 L236 L259 | L156 L157 L158 L258 | L150 L151 L152 L259 | L252 L253 L254 L258 | L246 L247 L248 L259 | L168 L169 L170 L258 | L162 L163 L164 L259 | L204 L205 L206 L258 | L198 L199 L200 L259 | L96 L97 L98 L258 | L90 L91 L92 L259 | L84 L85 L86 L258 | L78 L79 L80 L259 | L72 L73 L74 L258 | L66 L67 L68 L259 bodies 1
sketch "Sketch7" plane through (0, 10, 0) normal (0, 1, 0) x (-1, 0, 0)
  arc A0 (-5.0797, 0) -> (-2.1135, 2.5506) centre (-5.0797, 3) ccw
  line L0 (-2.1135, 2.5506) -> (-0.5226, 13.0506)
  arc A1 (-0.5226, 13.0506) -> (-3.4888, 16.5) centre (-3.4888, 13.5) ccw
  line L1 (-3.4888, 16.5) -> (-44.1, 16.5)
  arc A2 (-44.1, 16.5) -> (-47.1, 13.5) centre (-44.1, 13.5) ccw
  line L2 (-47.1, 13.5) -> (-47.1, 3)
  arc A3 (-47.1, 3) -> (-44.1, 0) centre (-44.1, 3) ccw
  line L3 (-44.1, 0) -> (-5.0797, 0)
  line L4 (-26.405, 10.29) -> (-26.405, 11.29)
  line L5 (-26.405, 11.29) -> (-24.005, 11.29)
  line L6 (-24.005, 11.29) -> (-24.005, 10.29)
  line L7 (-24.005, 10.29) -> (-26.405, 10.29)
  line L8 (-22.595, 10.29) -> (-22.595, 11.29)
  line L9 (-22.595, 11.29) -> (-20.195, 11.29)
  line L10 (-20.195, 11.29) -> (-20.195, 10.29)
  line L11 (-20.195, 10.29) -> (-22.595, 10.29)
  line L12 (-11.165, 10.29) -> (-11.165, 11.29)
  line L13 (-11.165, 11.29) -> (-8.765, 11.29)
  line L14 (-8.765, 11.29) -> (-8.765, 10.29)
  line L15 (-8.765, 10.29) -> (-11.165, 10.29)
  line L16 (-39.245, 11.29) -> (-39.245, 10.29)
  line L17 (-39.245, 10.29) -> (-41.645, 10.29)
  line L18 (-41.645, 10.29) -> (-41.645, 11.29)
  line L19 (-41.645, 11.29) -> (-39.245, 11.29)
  line L20 (-37.34, 6.21) -> (-37.34, 5.21)
  line L21 (-37.34, 5.21) -> (-39.74, 5.21)
  line L22 (-39.74, 5.21) -> (-39.74, 6.21)
  line L23 (-39.74, 6.21) -> (-37.34, 6.21)
  line L24 (-3.05, 6.21) -> (-3.05, 5.21)
  line L25 (-3.05, 5.21) -> (-5.45, 5.21)
  line L26 (-5.45, 5.21) -> (-5.45, 6.21)
  line L27 (-5.45, 6.21) -> (-3.05, 6.21)
  line L28 (-6.86, 6.21) -> (-6.86, 5.21)
  line L29 (-6.86, 5.21) -> (-9.26, 5.21)
  line L30 (-9.26, 5.21) -> (-9.26, 6.21)
  line L31 (-9.26, 6.21) -> (-6.86, 6.21)
  line L32 (-10.67, 6.21) -> (-10.67, 5.21)
  line L33 (-10.67, 5.21) -> (-13.07, 5.21)
  line L34 (-13.07, 5.21) -> (-13.07, 6.21)
  line L35 (-13.07, 6.21) -> (-10.67, 6.21)
  line L36 (-30.215, 10.29) -> (-30.215, 11.29)
  line L37 (-30.215, 11.29) -> (-27.815, 11.29)
  line L38 (-27.815, 11.29) -> (-27.815, 10.29)
  line L39 (-27.815, 10.29) -> (-30.215, 10.29)
  line L40 (-18.785, 10.29) -> (-18.785, 11.29)
  line L41 (-18.785, 11.29) -> (-16.385, 11.29)
  line L42 (-16.385, 11.29) -> (-16.385, 10.29)
  line L43 (-16.385, 10.29) -> (-18.785, 10.29)
  line L44 (-14.975, 10.29) -> (-14.975, 11.29)
  line L45 (-14.975, 11.29) -> (-12.575, 11.29)
  line L46 (-12.575, 11.29) -> (-12.575, 10.29)
  line L47 (-12.575, 10.29) -> (-14.975, 10.29)
  line L48 (-34.025, 10.29) -> (-34.025, 11.29)
  line L49 (-34.025, 11.29) -> (-31.625, 11.29)
  line L50 (-31.625, 11.29) -> (-31.625, 10.29)
  line L51 (-31.625, 10.29) -> (-34.025, 10.29)
  line L52 (-25.91, 6.21) -> (-25.91, 5.21)
  line L53 (-25.91, 5.21) -> (-28.31, 5.21)
  line L54 (-28.31, 5.21) -> (-28.31, 6.21)
  line L55 (-28.31, 6.21) -> (-25.91, 6.21)
  line L56 (-18.29, 6.21) -> (-18.29, 5.21)
  line L57 (-18.29, 5.21) -> (-20.69, 5.21)
  line L58 (-20.69, 5.21) -> (-20.69, 6.21)
  line L59 (-20.69, 6.21) -> (-18.29, 6.21)
  line L60 (-33.53, 6.21) -> (-33.53, 5.21)
  line L61 (-33.53, 5.21) -> (-35.93, 5.21)
  line L62 (-35.93, 5.21) -> (-35.93, 6.21)
  line L63 (-35.93, 6.21) -> (-33.53, 6.21)
  line L64 (-41.15, 6.21) -> (-41.15, 5.21)
  line L65 (-41.15, 5.21) -> (-43.55, 5.21)
  line L66 (-43.55, 5.21) -> (-43.55, 6.21)
  line L67 (-43.55, 6.21) -> (-41.15, 6.21)
  line L68 (-14.48, 6.21) -> (-14.48, 5.21)
  line L69 (-14.48, 5.21) -> (-16.88, 5.21)
  line L70 (-16.88, 5.21) -> (-16.88, 6.21)
  line L71 (-16.88, 6.21) -> (-14.48, 6.21)
  line L72 (-37.835, 10.29) -> (-37.835, 11.29)
  line L73 (-37.835, 11.29) -> (-35.435, 11.29)
  line L74 (-35.435, 11.29) -> (-35.435, 10.29)
  line L75 (-35.435, 10.29) -> (-37.835, 10.29)
  line L76 (-7.355, 10.29) -> (-7.355, 11.29)
  line L77 (-7.355, 11.29) -> (-4.955, 11.29)
  line L78 (-4.955, 11.29) -> (-4.955, 10.29)
  line L79 (-4.955, 10.29) -> (-7.355, 10.29)
  line L80 (-29.72, 6.21) -> (-29.72, 5.21)
  line L81 (-29.72, 5.21) -> (-32.12, 5.21)
  line L82 (-32.12, 5.21) -> (-32.12, 6.21)
  line L83 (-32.12, 6.21) -> (-29.72, 6.21)
  line L84 (-22.1, 6.21) -> (-22.1, 5.21)
  line L85 (-22.1, 5.21) -> (-24.5, 5.21)
  line L86 (-24.5, 5.21) -> (-24.5, 6.21)
  line L87 (-24.5, 6.21) -> (-22.1, 6.21)
  line L88 (-47.1, 8.25) -> (-59, 8.25) construction
  line L89 (-47.1, 8.25) -> (6.5921, 8.25) construction
  line L90 (-47.1, 12.35) -> (-50.7944, 12.35)
  line L91 (-50.7944, 12.35) -> (-50.7944, 4.15)
  line L92 (-50.7944, 4.15) -> (-47.1, 4.15)
  line L93 (-0.6288, 12.35) -> (3.2056, 12.35)
  line L94 (3.2056, 12.35) -> (3.2056, 4.15)
  line L95 (3.2056, 4.15) -> (-1.8712, 4.15)
  line L96 (-23.7944, 16.5) -> (-23.7944, 0) construction
  line L97 (-47.1, 10.35) -> (-49.7944, 10.35)
  line L98 (-49.7944, 10.35) -> (-49.7944, 6.15)
  line L99 (-49.7944, 6.15) -> (-47.1, 6.15)
  line L100 (-0.4884, 10.35) -> (2.2056, 10.35)
  line L101 (2.2056, 10.35) -> (2.2056, 6.15)
  line L102 (2.2056, 6.15) -> (-1.8712, 6.15)
  line L103 (-0.4884, 10.35) -> (-0.4884, 6.15)
  line L104 (2.7056, 4.15) -> (2.7056, -6)
  line L105 (1.2056, -1.7) -> (1.2056, 4.15)
  line L106 (2.7056, -6) -> (0.2056, -1.7)
  line L107 (0.2056, -1.7) -> (1.2056, -1.7)
  line L108 (-50.2944, 4.15) -> (-50.2944, -6)
  line L109 (-50.2944, -6) -> (-47.7944, -1.7)
  line L110 (-47.7944, -1.7) -> (-48.7944, -1.7)
  line L111 (-48.7944, -1.7) -> (-48.7944, 4.15)
  dimension "d50" = 54
  dimension "d51" = 8.2
  dimension "d52" = 8.2
  dimension "d55" = 6
  dimension "d57" = 1.5
  dimension "d59" = 1.5
  dimension "d60" = 6
  dimension "d61" = 1
  dimension "d65" = 50
  dimension "d67" = 1
  dimension "d68" = 2
  dimension "d69" = 2
  dimension "d70" = 1
  dimension "d71" = 2
  dimension "d72" = 2
  dimension "d73" = 2.694
  dimension "d175" = 1.7
  constraint midpoint L2 L88.start
  constraint perpendicular L2 L88
  constraint horizontal L90
  constraint perpendicular L90 L91
  constraint coincident L2 L92.end
  constraint perpendicular L2 L92
  constraint coincident L0 L93.start
  constraint perpendicular L78 L93
  constraint perpendicular L25 L94
  constraint coincident L0 L95.end
  constraint perpendicular L24 L95
  constraint midpoint L1 L96.start
  constraint coincident L3 L96.end
  constraint perpendicular L3 L96
  constraint symmetric L91 L94 L96
  constraint symmetric L88 L90 L92
  constraint coincident L102 L103.end
  constraint perpendicular L102 L103
  constraint coincident L95 L104.start
  constraint perpendicular L95 L104
  constraint coincident L95 L105.end
  constraint perpendicular L95 L105
  constraint perpendicular L105 L107
  constraint coincident L92 L108.start
  constraint perpendicular L92 L108
  constraint perpendicular L92 L111
  constraint coincident L92 L111.end
  constraint equal L105 L111
  constraint equal L107 L110
  constraint perpendicular L110 L111
  constraint parallel L93 L100
  constraint parallel L94 L101
  constraint parallel L95 L102
  constraint parallel L90 L97
  constraint parallel L91 L98
  constraint parallel L92 L99
  constraint symmetric L96 L105 L111
  measures "d50" distance of L91 L94
  measures "d51" distance of L90.end L91.end
  measures "d52" distance of L93.end L94.end
  measures "d55" distance of L3 L104.end
  measures "d57" distance of L104 L105
  measures "d59" distance of L108 L111
  measures "d60" distance of L3 L108.end
  measures "d61" distance of L109.end L110.end
  measures "d65" distance of L105 L111
  measures "d67" distance of L94 L101
  measures "d68" distance of L93 L100
  measures "d69" distance of L95 L102
  measures "d70" distance of L91 L98
  measures "d71" distance of L90 L97
  measures "d72" distance of L92 L99
  measures "d73" distance of L100.start L100.end
  measures "d175" distance of A3.end L110
extrude "Extrude7" add sketch "Sketch7" against normal blind 3.3 contours L0 L93 L94 L95 | L95 L104 L105 L106 L107 | L2 L90 L91 L92 L97 L98 L99 | L92 L108 L109 L110 L111 bodies 1